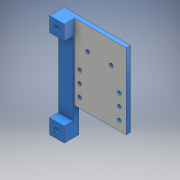
# Autodesk Inventor part: Support AX12
Saved by Autodesk Inventor 2018 (Build 220112000, 112)
## iProperties
Part Number: Support AX12
Material: Générique
Document SubType Name: Modeling
Designer: sasha
Density: 1 g/cm^3
Appearance: Par défaut
Author: sasha
Autodesk Inventor part; units mm, degrees
ref_plane "YZ Plane" through (0, 0, 0) normal (1, 0, 0) x (0, 1, 0)
ref_plane "XZ Plane" through (0, 0, 0) normal (0, 1, 0) x (-1, 0, 0)
ref_plane "XY Plane" through (0, 0, 0) normal (0, 0, 1) x (1, 0, 0)
sketch "Esquisse1" plane through (0, 0, 0) normal (0, 1, 0) x (-1, 0, 0)
  line L0 (0, 0) -> (35, 0)
  line L1 (35, 0) -> (35, -25)
  line L2 (35, -25) -> (0, -25) construction
  line L3 (0, -25) -> (0, 0) construction
  line L4 (35, 0) -> (45, 0)
  line L5 (45, 0) -> (45, -70)
  line L6 (45, -70) -> (35, -70)
  line L7 (35, -70) -> (35, 0)
  dimension "d0" = 25
  dimension "d1" = 35
  dimension "d2" = 10
  dimension "d3" = 70
  constraints: 16 end point, 4 parallel, 2 horizontal, 2 perpendicular
  measures "d0" distance of L0.end L1.end
  measures "d1" distance of L1.end L2.end
  measures "d2" distance of L5.end L6.end
  measures "d3" distance of L4.end L5.end
extrude "Extrusion1" add sketch "Esquisse1" along normal blind 10
sketch "Esquisse3" plane through (0, 10, 0) normal (0, 1, 0) x (1, 0, 0)
  line L0 (-35, 0) -> (0, 0)
  line L1 (0, 0) -> (0, 51.22)
  line L2 (0, 51.22) -> (-35, 51.22)
  line L3 (-35, 51.22) -> (-35, 0)
  line L4 (-35, 0) -> (-35, 70) projected
  line L5 (-45, 0) -> (-35, 0) projected
  point P0 (0, 0)
  dimension "d11" = 35
  dimension "d12" = 51.22
  constraints: 8 end point, 2 collinear, 2 parallel, 1 horizontal, 1 perpendicular
  measures "d11" distance of L0.start L0.end
  measures "d12" distance of L2.end L0.start
extrude "Extrusion3" add sketch "Esquisse3" against normal blind 3
sketch "Esquisse7" plane through (-35, 0, 0) normal (1, 0, 0) x (0, 0, -1)
  line L0 (10, 0) -> (60, 0)
  line L1 (60, 0) -> (60, 6)
  line L2 (60, 6) -> (10, 6)
  line L3 (10, 6) -> (10, 0)
  line L4 (70, 0) -> (0, 0) projected
  line L5 (51.22, 7) -> (0, 7) projected
  line L6 (70, 0) -> (70, 10) projected
  line L7 (0, 0) -> (0, 7) projected
  dimension "d23" = 1
  dimension "d24" = 10
  dimension "d25" = 10
  constraints: 8 end point, 2 parallel, 1 collinear, 1 horizontal, 1 perpendicular
  measures "d23" distance between parallel lines of L5 L2
  measures "d24" distance between parallel lines of L6 L1
  measures "d25" distance between parallel lines of L7 L3
extrude "Extrusion6" cut sketch "Esquisse7" against normal up to surface (10 mm away)
sketch "Esquisse8" plane through (0, 10, 0) normal (0, 1, 0) x (1, 0, 0)
  line L0 (-45, 70) -> (-45, 0) projected
  line L1 (-45, 5) -> (0, 5)
  line L2 (0, 51.22) -> (0, 0) projected
  line L3 (-45, 0) -> (0, 0) projected
  line L4 (-35.3134, 65) -> (-45, 65)
  line L5 (-35, 70) -> (-45, 70) projected
  line L6 (-40, 70) -> (-40, 0)
  point P0 (0, 0)
  point P1 (-40.1567, 5)
  point P2 (-40, 65)
  dimension "d28" = 5
  dimension "d29" = 5
  constraints: 7 point on line, 6 end point, 2 horizontal, 1 midpoint, 1 perpendicular
  measures "d28" distance between parallel lines of L3 L1
  measures "d29" distance between parallel lines of L4 L5
hole "Perçage1" at (-40.1567, 10, -5) at (-40, 10, -65) direction (0, -1, 0) diameter 3.4 end through all
sketch "Esquisse9" plane through (0, 10, 0) normal (0, 1, 0) x (1, 0, 0)
  line L0 (-18, 0) -> (-18, 24.9176)
  line L1 (-45, 70) -> (-45, 0) projected
  line L2 (0, 0) -> (-35, 0) projected
  line L3 (-31.5, 0) -> (-31.5, 51.22)
  line L4 (-45, 0) -> (0, 0) projected
  line L5 (-4.5, 0) -> (-4.5, 51.22)
  line L6 (-35, 51.22) -> (0, 51.22) projected
  line L7 (-35, 51.22) -> (-1, 51.22)
  line L8 (-35, 70) -> (-45, 70) projected
  line L9 (-45, 15.22) -> (0, 15.22)
  line L10 (-35, 44.72) -> (0, 44.72)
  line L11 (-18, 24.9176) -> (-18, 51.22)
  circle A0 centre (-18, 51.22) radius 10
  line L12 (-31.5, 36.72) -> (-4.5, 36.72)
  line L13 (-31.5, 28.72) -> (-4.5, 28.72)
  point P0 (-4.5, 44.72)
  point P1 (-31.5, 44.72)
  point P2 (-4.5, 44.72)
  point P3 (-26, 15.22)
  point P4 (-10, 15.22)
  dimension "d37" = 27
  dimension "d38" = 13.5
  dimension "d39" = 13.5
  dimension "d40" = 18.78
  dimension "d41" = 36
  dimension "d42" = 6.5
  dimension "d43" = 20
  dimension "d45" = 8
  dimension "d46" = 8
  dimension "d59" = 8
  dimension "d60" = 8
  constraints: 18 end point, 15 point on line, 6 coincident, 4 perpendicular, 3 horizontal, 2 vertical, 1 centre point, 1 midpoint
  measures "d37" distance between parallel lines of L1 L0
  measures "d38" distance between parallel lines of L3 L0
  measures "d39" distance between parallel lines of L5 L0
  measures "d40" distance between parallel lines of L7 L8
  measures "d41" distance between parallel lines of L7 L9
  measures "d42" distance between parallel lines of L7 L10
  measures "d43" diameter of A0
  measures "d45" distance from line of point (-26, 15.22) L0
  measures "d46" distance from line of L0 point (-10, 15.22)
  measures "d59" distance between parallel lines of L10 L12
  measures "d60" distance between parallel lines of L12 L13
hole "Perçage2" at (-26, 10, -15.22) at (-10, 10, -15.22) at (-31.5, 10, -44.72) at (-4.5, 10, -44.72) at (-31.5, 10, -36.72) at (-4.5, 10, -36.72) at (-31.5, 10, -28.72) at (-4.5, 10, -28.72) direction (0, -1, 0) diameter 2.5 end through all
sketch "Esquisse18" plane through (0, 10, 0) normal (0, 1, 0) x (1, 0, 0)
  circle A0 centre (-40, 65) radius 1.7 projected
  circle A1 centre (-40.1567, 5) radius 1.7 projected
  point P0 (0, 0)
  constraints: 2 coincident
hole "Perçage5" at (-40.1567, 10, -5) at (-40, 10, -65) direction (0, -1, 0) diameter 6.5 depth 2
